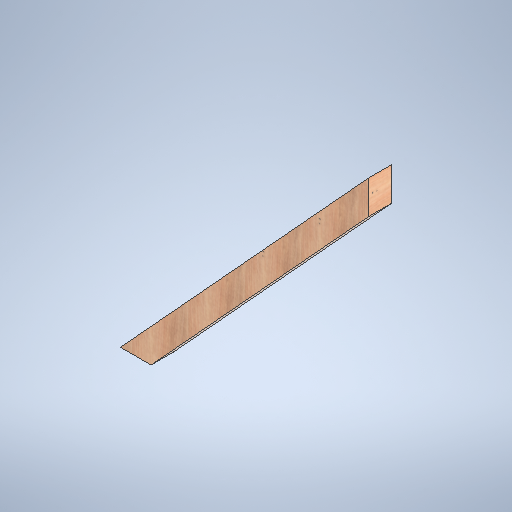
# Autodesk Inventor part: 4x4xidkanymore
Saved by Autodesk Inventor 2025 (Build 290162000, 162)
## iProperties
Created: 2024-08-18
Part Number: 4x4xidkanymore
Material: Generic
Document SubType Name: Modeling
Designer: Cupri
Density: 1 g/cm^3
Appearance: Default
Author: Cupri
Autodesk Inventor part; units mm, degrees
ref_plane "YZ Plane" through (0, 0, 0) normal (1, 0, 0) x (0, 1, 0)
ref_plane "XZ Plane" through (0, 0, 0) normal (0, 1, 0) x (-1, 0, 0)
ref_plane "XY Plane" through (0, 0, 0) normal (0, 0, 1) x (1, 0, 0)
sketch "Sketch1" plane through (0, 0, 0) normal (0, 0, 1) x (1, 0, 0)
  line L0 (-592.8645, -609.8015) -> (-491.2645, -609.8015)
  line L1 (524.7355, 609.3985) -> (-592.8645, -609.8015)
  line L2 (524.7355, 609.3985) -> (599.6304, 540.7448) construction
  line L3 (524.7355, 459.0414) -> (-455.0371, -609.8015)
  line L4 (-592.8645, -609.8015) -> (-455.0371, -609.8015)
  line L5 (-592.8645, -609.8015) -> (-455.0371, -609.8015)
  line L6 (524.7355, 609.3985) -> (524.7355, 459.0414)
  point P0 (0, 0)
  dimension "d0" = 101.6
  constraints: 14 end point, 2 perpendicular, 1 collinear, 1 vertical
  measures "d0" distance of L1.start L2.end
extrude "Extrusion1" add sketch "Sketch1" along normal blind 101.6
body "Solid1"
